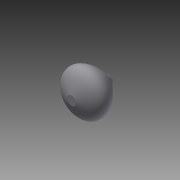
# Autodesk Inventor part: mallet2
Saved by Autodesk Inventor 2015 (Build 190159000, 159)
## iProperties
Created: 2014-07-11
Part Number: mallet2
Material: Generic
Document SubType Name: Modeling
Designer: shohei
Density: 1 g/cm^3
Appearance: Default
Mass: 43.4398 g
Surface Area: 62.0142 cm^2
Volume: 43.4398 cm^3
Author: shohei
Autodesk Inventor part; units mm, degrees
ref_plane "YZ Plane" through (0, 0, 0) normal (1, 0, 0) x (0, 1, 0)
ref_plane "XZ Plane" through (0, 0, 0) normal (0, 1, 0) x (-1, 0, 0)
ref_plane "XY Plane" through (0, 0, 0) normal (0, 0, 1) x (1, 0, 0)
sketch "Sketch1" plane through (0, 0, 0) normal (0, 0, 1) x (1, 0, 0)
  spline S0 degree 3 poles (-5, 0) (-46.3733, 12.8628) (-8.9091, 34.1083) (-5, 41) knots 0 0 0 0 1 1 1 1
  line L0 (-5, 41) -> (-5, 41)
  line L1 (-5, 41) -> (0, 41)
  line L2 (0, -9.4119) -> (0, 53.3926) projected
  line L3 (-5, 0) -> (0, 0)
  line L4 (0, 41) -> (0, 0)
  line L5 (-34.2276, 0) -> (9.5702, 0) projected
  point P0 (-24, 18)
  point P1 (-13, 33)
  dimension "d0" = 5
  dimension "d1" = 5
  dimension "d7" = 24
  dimension "d8" = 13
  dimension "d9" = 18
  dimension "d10" = 15
  dimension "d11" = 8
  dimension "d12" = 0
  constraints: 8 end point, 2 perpendicular, 1 horizontal, 1 vertical, 5 other
  measures "d0" distance between parallel lines of L2 L0
  measures "d1" distance from line of L2 point (-5, 0)
  measures "d7" distance from line of L2 point (-24, 18)
  measures "d8" distance from line of L2 point (-13, 33)
  measures "d9" distance from line of L5 point (-24, 18)
  measures "d10" vertical distance of point (-24, 18) point (-13, 33)
  measures "d11" horizontal distance of L0.start point (-13, 33)
  measures "d12" distance from line of L0.start L1
revolve "Revolution1" add sketch "Sketch1" angle 360 about axis through (0, -10, 0) along (0, 1, 0)
sketch "Sketch3" plane through (0, 41, 0) normal (0, 1, 0) x (1, 0, 0)
  circle A0 centre (0, 0) radius 1.5
  dimension "d4" = 3
  constraints: 1 centre point, 1 coincident
  measures "d4" diameter of A0
extrude "Extrusion1" cut sketch "Sketch3" against normal blind 5
body "Solid1"
